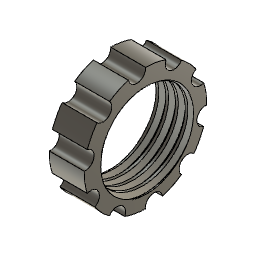
Nut (Autodesk Fusion 360 design; units mm, degrees)
Autodesk Fusion 360 part; units mm, degrees
sketch "Sketch1" plane through (0, 0, 0) normal (1, 0, 0) x (0, 1, 0)
  circle A0 centre (0, 0) radius 8.89
  circle A1 centre (0, 0) radius 2.9633
  dimension "d16" = 17.78
  constraint coincident A0.centre A1.centre
  constraint concentric A0 A1
  measures "d16" diameter of A0
extrude "Extrude5" add sketch "Sketch1" along normal blind 5.08
thread "Thread8" "ANSI Unified Screw Threads 0.5625 9/16-18 UNF 2B" major diameter 14.2875 minor diameter 12.9159 pitch 1.4111 angle 60 modelled right hand crest width 0.3991 on face at (3.3867, 2.9596, -0.1477) crest through (0.3528, 6.4579, 0)
cylinder "CylinderPrimitive1" cut diameter 2.54 height 7.62 placed x (0, 0, -1) y (0, 1, 0) z (1, 0, 0) at (0, 6.1642, -6.3705)
pattern_circular "C-Pattern1" count 10 over 360 about axis through (1.75, 0, 0) along (1, 0, 0) of "CylinderPrimitive1"
scale "Scale1" factor 1.03 about (5.08, -2.489, 8.5344) bodies 1
scale "Scale2" factor 1.02 about (5.08, 7.6427, 4.8986) bodies 1
